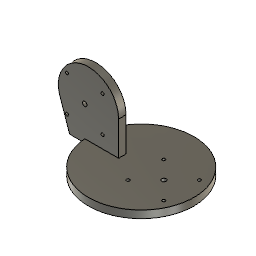
link1 (Autodesk Fusion 360 design; units mm, degrees)
part number: 2025-12-13-21-49-02-726
Autodesk Fusion 360 part; units mm, degrees
sketch "Sketch1" plane through (0, 0, 0) normal (0, 0, 1) x (1, 0, 0)
  circle A0 centre (0, 0) radius 70
  dimension "d1" = 140
  constraint coincident A0.centre origin
  measures "d1" diameter of A0
extrude "Extrude1" add sketch "Sketch1" along normal blind 10
sketch "Sketch2" plane through (0, 0, 0) normal (0, 0, -1) x (1, 0, 0)
  circle A0 centre (0, 0) radius 70
  circle A1 centre (0, 0) radius 65
  dimension "d4" = -5
extrude "Extrude2" add sketch "Sketch2" along normal blind 3 contours A1
sketch "Sketch3" plane through (0, 0, 0) normal (0, 1, 0) x (1, 0, 0)
  line L0 (-25, -55) -> (-25, -5)
  line L1 (-25, -5) -> (-90, -5)
  line L2 (-90, -5) -> (-103.8281, -45.3888)
  arc A0 (-103.8281, -45.3888) -> (-25, -55) centre (-65, -55) ccw
  dimension "d7" = 50
  dimension "d8" = 65
  dimension "d9" = 40
  dimension "d12" = 5
  dimension "d14" = 25
  constraint vertical L0
  constraint perpendicular L0 L1
  constraint tangent L0 A0
  measures "d7" distance of L0.start L0.end
  measures "d8" distance of L0.end L1.end
  measures "d9" radius of A0
  measures "d12" distance of origin L1
  measures "d14" horizontal distance of origin L0.end
extrude "Extrude3" add sketch "Sketch3" along normal mid plane 10
sketch "Sketch4" plane through (0, 0, 10) normal (0, 0, 1) x (-1, 0, 0)
  line L0 (69.8212, -5) -> (25, -5)
  line L1 (25, -5) -> (25, 5)
  line L2 (25, 5) -> (69.8212, 5)
  arc A0 (69.8212, 5) -> (69.8212, -5) centre (0, 0) ccw
  line L3 (-6.378, 23.622) -> (-53.622, 23.622)
  line L4 (-53.622, 23.622) -> (-53.622, -23.622)
  line L5 (-53.622, -23.622) -> (-6.378, -23.622)
  line L6 (-6.378, -23.622) -> (-6.378, 23.622)
  line L7 (-6.378, 23.622) -> (-53.622, -23.622) construction
  line L8 (-53.622, 23.622) -> (-6.378, -23.622) construction
  point P0 (-30, 0)
  dimension "d17" = 47.244
  dimension "d18" = 47.244
  dimension "d20" = 30
  constraint horizontal L3
  constraint perpendicular L3 L4
  constraint parallel L3 L5
  constraint parallel L4 L6
  constraint coincident L7 P0
  constraint coincident L8 P0
  constraint horizontal A0.centre P0
  measures "d17" distance of L3.end L4.end
  measures "d18" distance of L4.end L5.end
  measures "d20" distance of A0.centre P0
hole "Hole1" at (6.378, 23.622, 10) at (53.622, 23.622, 10) at (53.622, -23.622, 10) at (6.378, -23.622, 10) direction (0, 0, -1) diameter 4 depth 15 tip angle 118
hole "Hole2" at (30, 0, 10) direction (0, 0, -1) diameter 6 depth 15 tip angle 118
sketch "Sketch5" plane through (0, -5, 0) normal (0, -1, 0) x (1, 0, 0)
  line L0 (-69.8212, 10) -> (-25, 10)
  line L1 (-25, 10) -> (-25, 55)
  arc A0 (-25, 55) -> (-103.8281, 45.3888) centre (-65, 55) ccw
  line L2 (-103.8281, 45.3888) -> (-90, 5)
  line L3 (-90, 5) -> (-69.8212, 5)
  line L4 (-69.8212, 5) -> (-69.8212, 10)
  line L5 (-93.4432, 73.622) -> (-46.1992, 73.622)
  line L6 (-46.1992, 73.622) -> (-46.1992, 26.378)
  line L7 (-46.1992, 26.378) -> (-93.4432, 26.378)
  line L8 (-93.4432, 26.378) -> (-93.4432, 73.622)
  line L9 (-93.4432, 73.622) -> (-46.1992, 26.378) construction
  line L10 (-46.1992, 73.622) -> (-93.4432, 26.378) construction
  point P0 (-69.8212, 50)
  dimension "d27" = 47.244
  dimension "d28" = 47.244
  dimension "d30" = 45
  constraint horizontal L5
  constraint perpendicular L5 L6
  constraint parallel L5 L7
  constraint parallel L6 L8
  constraint coincident L9 P0
  constraint coincident L10 P0
  constraint vertical L3.end P0
  measures "d27" distance of L5.end L6.end
  measures "d28" distance of L6.end L7.end
  measures "d30" distance of L3 P0
hole "Hole3" at (-93.4432, -5, 73.622) at (-46.1992, -5, 73.622) at (-93.4432, -5, 26.378) at (-46.1992, -5, 26.378) direction (0, 1, 0) diameter 4 depth 15 tip angle 118
hole "Hole4" at (-69.8212, -5, 50) direction (0, 1, 0) diameter 6 depth 15 tip angle 118
